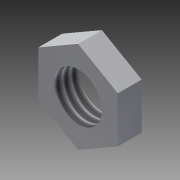
# Autodesk Inventor part: M3 Nut Nylon
Saved by Autodesk Inventor 2015 (Build 190159000, 159)
## iProperties
Created: 2016-02-19
Part Number: M3 Nut Nylon
Material: Nylon 6
Document SubType Name: Modeling
Designer: 23902
Density: 1.12 g/cm^3
Appearance: Nylon 6
Mass: 0.0244978 g
Surface Area: 0.69282 cm^2
Volume: 0.0218731 cm^3
Author: 23902
Autodesk Inventor part; units mm, degrees
ref_plane "YZ Plane" through (0, 0, 0) normal (1, 0, 0) x (0, 1, 0)
ref_plane "XZ Plane" through (0, 0, 0) normal (0, 1, 0) x (-1, 0, 0)
ref_plane "XY Plane" through (0, 0, 0) normal (0, 0, 1) x (1, 0, 0)
sketch "Sketch1" plane through (0, 0, 0) normal (0, 1, 0) x (-1, 0, 0)
  circle A0 centre (0, 0) radius 1.5
  line L0 (0, -2.8868) -> (-2.5, -1.4434)
  line L1 (-2.5, -1.4434) -> (-2.5, 1.4434)
  line L2 (-2.5, 1.4434) -> (0, 2.8868)
  line L3 (0, 2.8868) -> (2.5, 1.4434)
  line L4 (2.5, 1.4434) -> (2.5, -1.4434)
  line L5 (2.5, -1.4434) -> (0, -2.8868)
  dimension "d0" = 3
  dimension "d1" = 5
  constraints: 12 end point, 2 coincident, 1 centre point, 13 other
  measures "d0" diameter of A0
  measures "d1" distance between parallel lines of L0 L3
extrude "Extrusion1" add sketch "Sketch1" along normal blind 1.5
thread "Thread1" size "M3x0.5" class "6H" standard "ANSI Metric M Profile" full length
body "Solid1"
